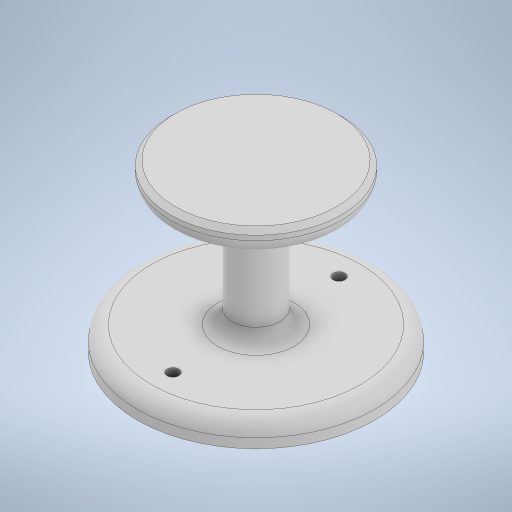
# Autodesk Inventor part: holding_socket
Saved by Autodesk Inventor 2023 (Build 270158000, 158)
## iProperties
Created: 2023-02-27
Part Number: holding_socket
Material: Generic
Document SubType Name: Modeling
Designer: maste
Density: 1 g/cm^3
Appearance: Default
Author: maste
Autodesk Inventor part; units mm, degrees
ref_plane "YZ Plane" through (0, 0, 0) normal (1, 0, 0) x (0, 1, 0)
ref_plane "XZ Plane" through (0, 0, 0) normal (0, 1, 0) x (-1, 0, 0)
ref_plane "XY Plane" through (0, 0, 0) normal (0, 0, 1) x (1, 0, 0)
sketch "Sketch2" plane through (0, 0, 0) normal (0, 0, 1) x (1, 0, 0)
  line L0 (0, 0) -> (25, 0)
  line L1 (0, 0) -> (0, 35)
  line L2 (0, 35) -> (18, 35)
  line L3 (18, 35) -> (18, 30)
  line L4 (18, 30) -> (5, 30)
  line L5 (5, 30) -> (5, 5)
  line L6 (5, 5) -> (25, 5)
  line L7 (25, 5) -> (25, 0)
  dimension "d3" = 25
  dimension "d4" = 35
  dimension "d5" = 18
  dimension "d6" = 5
  dimension "d23" = 5
  dimension "d24" = 25
  dimension "d26" = 5
  constraints: 16 end point, 6 perpendicular, 1 horizontal, 1 vertical
  measures "d3" distance of L0.start L0.end
  measures "d4" distance of L0.start L1.end
  measures "d5" distance of L1.end L2.end
  measures "d6" distance of L2.end L3.end
  measures "d23" distance of L6.end L0.end
  measures "d24" distance of L4.end L5.end
  measures "d26" distance between parallel lines of L1 L5
revolve "Revolution1" add sketch "Sketch2" angle 360 about axis through (0, 0, 0) along (0, 1, 0)
fillet "Fillet1" radius 3 3 edges at (-5, 5, 0) (-18, 30, 0) (-25, 5, 0)
chamfer "Chamfer1" distance 1 angle 45 1 edges at (-18, 35, 0)
sketch "Sketch3" plane through (0, 0, 0) normal (0, -1, 0) x (1, 0, 0)
  line L0 (0, 0) -> (0, -17.5)
  line L1 (0, 0) -> (0, 17.5)
  dimension "d14" = 17.5
  dimension "d15" = 17.5
  constraints: 4 end point, 2 coincident, 2 vertical
  measures "d14" distance of L0.start L0.end
  measures "d15" distance of L0.start L1.end
hole "Hole1" at (0, 0, 17.5) at (0, 0, -17.5) direction (0, 1, 0) diameter 2.5 depth 5 tip angle 118
fillet "Fillet2" radius 7 1 edges at (-5, 30, 0)
body "Solid2"
